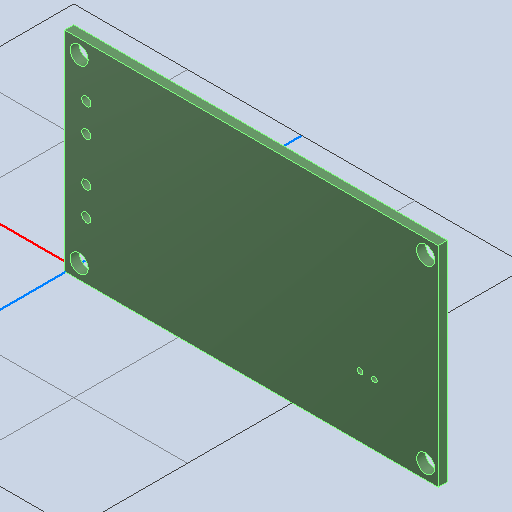
# Autodesk Inventor part: untitled.brdКонтур
Saved by Autodesk Inventor 2022 (Build 260153000, 153)
## iProperties
Created: 2023-03-06
Part Number: untitled.brdКонтур
Material: Типовые
Document SubType Name: Modeling
Designer: Иван Петров
Density: 1 g/cm^3
Appearance: Контур панели
Author: Иван Петров
Autodesk Inventor part; units mm, degrees
ref_plane "YZ Plane" through (0, 0, 0) normal (1, 0, 0) x (0, 1, 0)
ref_plane "XZ Plane" through (0, 0, 0) normal (0, 1, 0) x (-1, 0, 0)
ref_plane "XY Plane" through (0, 0, 0) normal (0, 0, 1) x (1, 0, 0)
sketch "Эскиз1" plane through (0, 0, 0) normal (0, 0, 1) x (1, 0, 0)
  line L0 (0, -7.62) -> (65.71, -7.62)
  line L1 (65.71, -7.62) -> (65.71, 29.2)
  line L2 (65.71, 29.2) -> (0, 29.2)
  line L3 (0, 29.2) -> (0, -7.62)
  circle A0 centre (3.81, 15.24) radius 0.8
  circle A1 centre (3.81, 20.24) radius 0.8
  circle A2 centre (3.81, 2.54) radius 0.8
  circle A3 centre (3.81, 7.54) radius 0.8
  circle A4 centre (51.94, 3.18) radius 0.5
  circle A5 centre (54.48, 3.18) radius 0.5
  circle A6 centre (2.54, 26.67) radius 1.6
  circle A7 centre (2.54, -5.08) radius 1.6
  circle A8 centre (63.5, -5.08) radius 1.6
  circle A9 centre (63.5, 26.67) radius 1.6
  constraints: 10 centre point, 8 end point
extrude "untitled.brdКонтур" add sketch "Эскиз1" along normal blind 1.6
